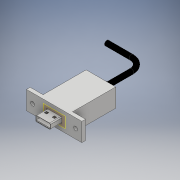
# Autodesk Inventor part: usb head
Saved by Autodesk Inventor 2018 (Build 220112000, 112)
## iProperties
Created: 2017-01-24
Part Number: usb head
Material: Generic
Document SubType Name: Modeling
Designer: shinezackery
Density: 1 g/cm^3
Appearance: Default
Author: shinezackery
Autodesk Inventor part; units mm, degrees
ref_plane "YZ Plane" through (0, 0, 0) normal (1, 0, 0) x (0, 1, 0)
ref_plane "XZ Plane" through (0, 0, 0) normal (0, 1, 0) x (-1, 0, 0)
ref_plane "XY Plane" through (0, 0, 0) normal (0, 0, 1) x (1, 0, 0)
sketch "Sketch1" plane through (0, 0, 0) normal (0, 0, 1) x (1, 0, 0)
  line L0 (0, 0) -> (16.16, 0)
  line L1 (16.16, 0) -> (16.16, 20.88)
  line L2 (16.16, 20.88) -> (13.48, 31.48)
  line L3 (13.48, 31.48) -> (2.68, 31.48)
  line L4 (2.68, 31.48) -> (0, 20.88)
  line L5 (0, 20.88) -> (0, 0)
  point P0 (8.08, 31.48)
  point P1 (8.08, 0)
  dimension "d2" = 16.16
  dimension "d3" = 20.88
  dimension "d4" = 10.8
  dimension "d5" = 10.6
  constraints: 12 end point, 2 horizontal, 2 midpoint, 2 vertical, 1 horizontal alignment, 1 vertical alignment
  measures "d2" distance of L0.start L0.end
  measures "d3" distance of L0.end L1.end
  measures "d4" distance of L2.end L3.end
  measures "d5" vertical distance of L1.end L2.end
extrude "Extrusion1" add sketch "Sketch1" along normal blind 8
chamfer "Chamfer1" distance 1 angle 45 8 edges at (16.16, 10.44, 8) (14.82, 26.18, 8) (14.82, 26.18, 0) (16.16, 10.44, 0) (0, 10.44, 0) (0, 10.44, 8) (1.34, 26.18, 0) (1.34, 26.18, 8)
fillet "Fillet1" radius 0.5 16 edges at (15.16, 10.3778, 8) (13.8043, 26.1178, 8) (14.82, 26.18, 7) (16.16, 10.44, 7) (16.16, 10.44, 1) (15.16, 10.3778, 0) (14.82, 26.18, 1) (13.8043, 26.1178, 0) (1.34, 26.18, 1) (2.3557, 26.1178, 0) (0, 10.44, 1) (1, 10.3778, 0) (1.34, 26.18, 7) (2.3557, 26.1178, 8) (1, 10.3778, 8) (0, 10.44, 7)
fillet "Fillet2" radius 3 7 edges at (0.0381, 20.8753, 6.9842) (0.5, 20.8178, 7.5) (1.0158, 20.7536, 7.9619) (0.0381, 20.8753, 1.0158) (0.5, 20.8178, 0.5) (1.0158, 20.7536, 0.0381) (0, 20.88, 4)
fillet "Fillet3" radius 3 7 edges at (16.1219, 20.8753, 6.9842) (15.66, 20.8178, 7.5) (15.1442, 20.7536, 7.9619) (16.1219, 20.8753, 1.0158) (15.66, 20.8178, 0.5) (15.1442, 20.7536, 0.0381) (16.16, 20.88, 4)
sketch "Sketch2" plane through (0, 0, 8) normal (0, 0, 1) x (1, 0, 0)
  line L0 (4.205, 2.3) -> (11.955, 2.3)
  line L1 (11.955, 2.3) -> (11.955, 17.2)
  line L2 (11.955, 17.2) -> (4.205, 17.2)
  line L3 (4.205, 17.2) -> (4.205, 2.3)
  line L4 (1.2071, 0) -> (14.9529, 0) projected
  point P0 (0, 0)
  point P1 (8.08, 0)
  point P2 (8.08, 2.3)
  dimension "d14" = 7.75
  dimension "d15" = 14.9
  dimension "d16" = 2.3
  constraints: 8 end point, 2 midpoint, 2 parallel, 1 horizontal, 1 perpendicular, 1 vertical alignment
  measures "d14" distance of L1.end L2.end
  measures "d15" distance of L0.end L1.end
  measures "d16" distance between parallel lines of L0 L4
extrude "Extrusion2" cut sketch "Sketch2" against normal blind 0.3
sketch "Sketch4" plane through (1.2071, 0, 0) normal (0, -1, 0) x (1, 0, 0)
  line L0 (0.8729, 1.75) -> (12.8729, 1.75)
  line L1 (12.8729, 1.75) -> (12.8729, 6.25)
  line L2 (12.8729, 6.25) -> (0.8729, 6.25)
  line L3 (0.8729, 6.25) -> (0.8729, 1.75)
  line L4 (0, 8) -> (13.7458, 8) projected
  line L5 (14.9529, 1.2071) -> (14.9529, 6.7929) projected
  point P0 (-1.2071, 0)
  point P1 (6.8729, 6.25)
  point P2 (6.8729, 8)
  point P3 (12.8729, 4)
  point P4 (14.9529, 4)
  dimension "d19" = 12
  dimension "d20" = 4.5
  constraints: 8 end point, 4 midpoint, 3 perpendicular, 1 horizontal, 1 horizontal alignment, 1 vertical alignment
  measures "d19" distance of L1.end L2.end
  measures "d20" distance of L0.end L1.end
extrude "Extrusion3" add sketch "Sketch4" along normal blind 12
fillet "Fillet4" radius 0.75 4 edges at (14.08, -6, 6.25) (14.08, -6, 1.75) (2.08, -6, 6.25) (2.08, -6, 1.75)
sketch "Sketch5" plane through (2.83, 0, 6.25) normal (0, 0, 1) x (1, 0, 0)
  line L0 (7.45, -7) -> (9.45, -7)
  line L1 (9.45, -7) -> (9.45, -5)
  line L2 (9.45, -5) -> (7.45, -5)
  line L3 (7.45, -5) -> (7.45, -7)
  line L4 (3.05, -7) -> (1.05, -7)
  line L5 (1.05, -7) -> (1.05, -5)
  line L6 (1.05, -5) -> (3.05, -5)
  line L7 (3.05, -5) -> (3.05, -7)
  line L8 (10.5, -12) -> (0, -12) projected
  line L9 (-1.6229, 0) -> (12.1229, 0) projected
  line L10 (11.25, -12) -> (11.25, 0) projected
  line L11 (-0.75, 0) -> (-0.75, -12) projected
  line L12 (0, 0) -> (10.5, 0) projected
  line L13 (5.6528, 0) -> (5.6528, -0.9812)
  line L14 (5.6528, -0.9812) -> (5.25, -0.9812)
  line L15 (5.25, -0.9812) -> (5.25, -8.4409)
  line L16 (5.25, -8.4409) -> (5.7498, -8.4409)
  line L17 (5.7498, -8.4409) -> (5.7498, -10.4572)
  line L18 (5.7498, -10.4572) -> (5.25, -10.4572)
  line L19 (5.25, -10.4572) -> (5.25, -12)
  point P0 (-2.83, 0)
  dimension "d24" = 5
  dimension "d25" = 5
  dimension "d26" = 2
  dimension "d27" = 2
  dimension "d28" = 1.8
  dimension "d29" = 1.8
  constraints: 30 end point, 8 perpendicular, 4 parallel, 4 point on line, 2 horizontal, 1 midpoint
  measures "d24" distance between parallel lines of L8 L0
  measures "d25" distance between parallel lines of L9 L2
  measures "d26" distance between parallel lines of L3 L1
  measures "d27" distance between parallel lines of L7 L5
  measures "d28" distance between parallel lines of L10 L1
  measures "d29" distance between parallel lines of L11 L5
extrude "Extrusion4" cut sketch "Sketch5" against normal blind 2.45
sketch "Sketch6" plane through (1.2071, -12, 0) normal (0, -1, 0) x (1, 0, 0)
  arc A0 (0.8729, 2.5) -> (1.6229, 1.75) centre (1.6229, 2.5) ccw projected
  line L0 (1.6229, 1.75) -> (12.1229, 1.75) projected
  arc A1 (12.1229, 1.75) -> (12.8729, 2.5) centre (12.1229, 2.5) ccw projected
  line L1 (12.8729, 2.5) -> (12.8729, 5.5) projected
  arc A2 (12.8729, 5.5) -> (12.1229, 6.25) centre (12.1229, 5.5) ccw projected
  line L2 (12.1229, 6.25) -> (1.6229, 6.25) projected
  arc A3 (1.6229, 6.25) -> (0.8729, 5.5) centre (1.6229, 5.5) ccw projected
  line L3 (0.8729, 5.5) -> (0.8729, 2.5) projected
  line L4 (1.6229, 5.95) -> (12.1229, 5.95)
  arc A4 (12.5729, 5.5) -> (12.1229, 5.95) centre (12.1229, 5.5) ccw
  line L5 (12.5729, 5.5) -> (12.5729, 2.5)
  arc A5 (12.1229, 2.05) -> (12.5729, 2.5) centre (12.1229, 2.5) ccw
  line L6 (12.1229, 2.05) -> (1.6229, 2.05)
  arc A6 (1.1729, 2.5) -> (1.6229, 2.05) centre (1.6229, 2.5) ccw
  line L7 (1.1729, 2.5) -> (1.1729, 5.5)
  arc A7 (1.6229, 5.95) -> (1.1729, 5.5) centre (1.6229, 5.5) ccw
  point P0 (-1.2071, 0)
  dimension "d32" = 0.3
  constraints: 8 end point, 8 point on circle, 4 centre point, 7 other
  measures "d32" distance between parallel lines of L2 L4
extrude "Extrusion5" cut sketch "Sketch6" against normal blind 0.2 contours L4 A4 L5 A5 L6 A6 L7 A7
sketch "Sketch7" plane through (1.2071, -11.8, 0) normal (0, -1, 0) x (1, 0, 0)
  line L0 (1.1729, 2.5) -> (1.1729, 5.5) projected
  line L1 (1.1739, 2.8515) -> (12.5698, 2.8515)
  line L2 (12.1229, 2.05) -> (1.6229, 2.05) projected
  arc A0 (1.6229, 5.95) -> (1.1729, 5.5) centre (1.6229, 5.5) ccw projected
  line L3 (1.6229, 5.95) -> (12.1229, 5.95) projected
  arc A1 (12.5729, 5.5) -> (12.1229, 5.95) centre (12.1229, 5.5) ccw projected
  line L4 (12.5729, 5.5) -> (12.5729, 2.5) projected
  line L5 (12.5719, 2.8515) -> (12.5719, 5.5)
  arc A2 (12.5719, 5.5) -> (12.1229, 5.949) centre (12.1229, 5.5) ccw
  line L6 (12.1229, 5.949) -> (1.6229, 5.949)
  arc A3 (1.6229, 5.949) -> (1.1739, 5.5) centre (1.6229, 5.5) ccw
  line L7 (1.1739, 5.5) -> (1.1739, 2.8515)
  line L8 (12.5698, 2.8515) -> (12.5719, 2.8515)
  point P0 (-1.2071, 0)
  dimension "d35" = 0.8015
  dimension "d36" = 0.001
  constraints: 10 end point, 4 point on circle, 2 centre point, 2 horizontal, 2 perpendicular, 1 point on line, 2 other
  measures "d35" distance between parallel lines of L2 L1
  measures "d36" distance between parallel lines of L6 L3
extrude "Extrusion6" cut sketch "Sketch7" against normal blind 9
sketch "Sketch8" plane through (0, 0, 7.7) normal (0, 0, 1) x (1, 0, 0)
  arc A0 (8.4073, 14.3419) -> (7.8073, 14.3289) centre (8.08, 15.6) ccw
  line L0 (4.205, 17.2) -> (11.955, 17.2) projected
  line L1 (7.8073, 4.1746) -> (7.3073, 4.1746)
  line L2 (8.4073, 4.1746) -> (8.9073, 4.1746)
  line L3 (7.3073, 4.1746) -> (8.08, 2.7708)
  line L4 (8.9073, 4.1746) -> (8.08, 2.7708)
  line L5 (8.4073, 12.3419) -> (9.9118, 11.2001)
  line L6 (8.6051, 12.7918) -> (10.4748, 11.3729)
  line L7 (11.955, 2.3) -> (4.205, 2.3) projected
  arc A1 (10.8703, 10.5763) -> (10.4748, 11.3729) centre (9.8703, 10.5763) ccw
  arc A2 (10.3073, 10.4035) -> (9.9118, 11.2001) centre (9.3073, 10.4035) ccw
  arc A3 (10.3073, 8.7573) -> (10.8703, 8.7573) centre (10.5888, 7.85) ccw
  line L8 (10.3073, 10.4035) -> (10.3073, 8.7573)
  line L9 (10.8703, 10.5763) -> (10.8703, 8.7573)
  line L10 (8.4073, 4.1746) -> (8.4073, 12.3419)
  line L11 (8.4073, 13.1901) -> (8.4073, 14.3419)
  arc A4 (8.4073, 13.1901) -> (8.6051, 12.7918) centre (8.9073, 13.1901) ccw
  line L12 (7.6001, 11.5555) -> (5.4489, 8.7573)
  line L13 (5.4489, 8.7573) -> (5.4489, 6.9)
  line L14 (6.0489, 6.9) -> (6.0489, 8.4673)
  line L15 (6.0489, 8.4673) -> (7.8073, 10.7545)
  line L16 (6.5489, 6.9) -> (6.5489, 5.4)
  line L17 (6.5489, 5.4) -> (4.9489, 5.4)
  line L18 (4.9489, 5.4) -> (4.9489, 6.9)
  line L19 (4.9489, 6.9) -> (5.4489, 6.9)
  line L20 (6.0489, 6.9) -> (6.5489, 6.9)
  line L21 (7.8073, 4.1746) -> (7.8073, 10.7545)
  line L22 (7.8073, 12.165) -> (7.8073, 14.3289)
  arc A5 (7.6001, 11.5555) -> (7.8073, 12.165) centre (6.8073, 12.165) ccw
  point P0 (0, 0)
  point P1 (8.08, 17.2)
  point P2 (10.3073, 10.9)
  constraints: 42 end point, 12 point on circle, 6 centre point, 6 parallel, 6 tangent, 6 vertical, 4 horizontal, 2 collinear, 2 perpendicular, 1 equal radius, 1 midpoint, 1 point on line, 1 vertical alignment
extrude "Extrusion7" add sketch "Sketch8" along normal blind 0.3
sketch "Sketch9" plane through (3.9251, 31.48, 0) normal (0, 1, 0) x (1, 0, 0)
  ellipse E0 centre (0, -7.5) end of major axis (-0.5157, -7.5) minor radius 0.5 (-0.3647, -7.8536) -> (0, -8) ccw projected
  line L0 (8.3098, -8) -> (0, -8) projected
  ellipse E1 centre (8.3098, -7.5) end of major axis (8.8256, -7.5) minor radius 0.5 (8.3098, -8) -> (8.6745, -7.8536) ccw projected
  line L1 (9.4039, -7.1464) -> (8.6745, -7.8536) projected
  ellipse E2 centre (9.0392, -6.7929) end of major axis (9.5549, -6.7929) minor radius 0.5 (9.4039, -7.1464) -> (9.5549, -6.7929) ccw projected
  line L2 (9.5549, -1.2071) -> (9.5549, -6.7929) projected
  ellipse E3 centre (9.0392, -1.2071) end of major axis (9.5549, -1.2071) minor radius 0.5 (9.5549, -1.2071) -> (9.4039, -0.8536) ccw projected
  line L3 (8.6745, -0.1464) -> (9.4039, -0.8536) projected
  ellipse E4 centre (8.3098, -0.5) end of major axis (8.8256, -0.5) minor radius 0.5 (8.6745, -0.1464) -> (8.3098, 0) ccw projected
  line L4 (8.3098, 0) -> (0, 0) projected
  ellipse E5 centre (0, -0.5) end of major axis (-0.5157, -0.5) minor radius 0.5 (0, 0) -> (-0.3647, -0.1464) ccw projected
  line L5 (-1.094, -0.8536) -> (-0.3647, -0.1464) projected
  ellipse E6 centre (-0.7294, -1.2071) end of major axis (-1.2451, -1.2071) minor radius 0.5 (-1.094, -0.8536) -> (-1.2451, -1.2071) ccw projected
  line L6 (-1.2451, -1.2071) -> (-1.2451, -6.7929) projected
  ellipse E7 centre (-0.7294, -6.7929) end of major axis (-1.2451, -6.7929) minor radius 0.5 (-1.2451, -6.7929) -> (-1.094, -7.1464) ccw projected
  line L7 (-0.3647, -7.8536) -> (-1.094, -7.1464) projected
  circle A0 centre (4.1549, -4) radius 3.7
  point P0 (-3.9251, 0)
  point P1 (4.1549, -8)
  point P2 (-1.2451, -4)
  dimension "d73" = 7.4
  constraints: 2 midpoint, 1 centre point, 1 horizontal alignment, 1 vertical alignment, 8 other
  measures "d73" diameter of A0
extrude "Extrusion8" add sketch "Sketch9" along normal blind 8.3 draft -5 contours A0
sketch "Sketch10" plane through (8.08, 39.78, 4) normal (0, 1, 0) x (1, 0, 0)
  circle A0 centre (0, 0) radius 1.95
  point P0 (-8.08, 4)
  dimension "d76" = 3.9
  constraints: 1 centre point
  measures "d76" diameter of A0
extrude "Extrusion9" add sketch "Sketch10" along normal blind 20
sketch "Sketch11" plane through (8.08, 59.78, 4) normal (0, 1, 0) x (1, 0, 0)
  circle A0 centre (0, 0) radius 1.95
  point P0 (-8.08, 4)
  constraints: 1 centre point
ref_plane "Work Plane1" through (0, 0, 4) normal (0, 0, 1) x (1, 0, 0)
sketch "Sketch12" plane through (0, 0, 4) normal (0, 0, 1) x (1, 0, 0)
  line L0 (10.03, 59.78) -> (6.13, 59.78) projected
  line L1 (8.08, 59.78) -> (8.08, 59.78)
  line L2 (-1.92, 69.78) -> (-21.92, 69.78)
  arc A0 (8.08, 59.78) -> (-1.92, 69.78) centre (-1.92, 59.78) ccw
  point P0 (0, 0)
  point P1 (8.08, 69.78)
  dimension "d79" = 10
  dimension "d80" = 30
  dimension "d81" = 10
  constraints: 4 end point, 2 point on circle, 2 point on line, 2 tangent, 1 centre point, 1 midpoint, 1 perpendicular, 1 vertical
  measures "d79" distance of L1.start point (8.08, 69.78)
  measures "d80" distance of point (8.08, 69.78) L2.end
  measures "d81" radius of A0
sweep "Sweep1" add profiles "Sketch11" path "Sketch12" path curves A0 L2
ref_plane "Work Plane2" through (1.2071, -3, 0) normal (0, -1, 0) x (1, 0, 0)
sketch "Sketch13" plane through (1.2071, -3, 0) normal (0, -1, 0) x (1, 0, 0)
  point P0 (-1.2071, 0)
sketch "Sketch14" plane through (1.2071, -3, 0) normal (0, -1, 0) x (1, 0, 0)
  line L0 (-1.2071, 1.2071) -> (-1.2071, 6.7929) projected
  line L1 (-1.2071, 4) -> (14.9529, 4)
  line L2 (14.9529, 6.7929) -> (14.9529, 1.2071) projected
  line L3 (6.8729, 4) -> (6.8729, 7.9846)
  line L4 (6.8729, 4) -> (6.8729, 0)
  line L5 (13.0729, 1.55) -> (0.6729, 1.55)
  line L6 (0.6729, 1.55) -> (0.6729, 6.45)
  line L7 (0.6729, 6.45) -> (13.0729, 6.45)
  line L8 (13.0729, 6.45) -> (13.0729, 1.55)
  line L9 (13.0729, 1.55) -> (0.6729, 6.45) construction
  line L10 (0.6729, 1.55) -> (13.0729, 6.45) construction
  line L11 (29.3729, -3.5) -> (-15.6271, -3.5)
  line L12 (-15.6271, -3.5) -> (-15.6271, 11.5)
  line L13 (-15.6271, 11.5) -> (29.3729, 11.5)
  line L14 (29.3729, 11.5) -> (29.3729, -3.5)
  line L15 (29.3729, -3.5) -> (-15.6271, 11.5) construction
  line L16 (-15.6271, -3.5) -> (29.3729, 11.5) construction
  point P0 (-1.2071, 0)
  dimension "d85" = 12.4
  dimension "d86" = 4.9
  dimension "d87" = 45
  dimension "d88" = 15
  constraints: 30 end point, 7 midpoint, 4 parallel, 2 horizontal, 2 perpendicular, 2 vertical
  measures "d85" distance of L6.end L7.end
  measures "d86" distance of L5.end L6.end
  measures "d87" distance of L12.end L13.end
  measures "d88" distance of L11.end L12.end
extrude "Extrusion10" add sketch "Sketch14" against normal blind 3
sketch "Sketch15" plane through (1.2071, 0, 0) normal (0, 1, 0) x (1, 0, 0)
  line L0 (-15.6271, -11.5) -> (29.3729, -11.5) projected
  line L1 (29.3729, 3.5) -> (-15.6271, 3.5) projected
  line L2 (29.3729, -11.5) -> (-15.6271, 3.5)
  line L3 (29.3729, 3.5) -> (-15.6271, -11.5)
  line L4 (-5.1271, 3.5) -> (18.8729, 3.5)
  line L5 (18.8729, 3.5) -> (18.8729, -11.5)
  line L6 (18.8729, -11.5) -> (-5.1271, -11.5)
  line L7 (-5.1271, -11.5) -> (-5.1271, 3.5)
  line L8 (-5.1271, 3.5) -> (18.8729, -11.5) construction
  line L9 (18.8729, 3.5) -> (-5.1271, -11.5) construction
  line L10 (-1.6271, 0.5) -> (15.3729, 0.5)
  line L11 (15.3729, 0.5) -> (15.3729, -8.5)
  line L12 (15.3729, -8.5) -> (-1.6271, -8.5)
  line L13 (-1.6271, -8.5) -> (-1.6271, 0.5)
  line L14 (-1.6271, 0.5) -> (15.3729, -8.5) construction
  line L15 (15.3729, 0.5) -> (-1.6271, -8.5) construction
  point P0 (-1.2071, 0)
  point P1 (6.8729, -4)
  dimension "d91" = 24
  dimension "d92" = 17
  dimension "d93" = 9
  constraints: 28 end point, 5 midpoint, 4 parallel, 2 horizontal, 2 perpendicular, 1 point on line
  measures "d91" distance of L5.end L6.end
  measures "d92" distance of L11.end L12.end
  measures "d93" distance of L10.end L11.end
extrude "Extrusion11" add sketch "Sketch15" along normal blind 35 contours L7 L3 L13 L12 L11 L2 L5 L0 | L7 L2 L13 L3 | L7 L1 L5 L3 L11 L10 L13 L2 | L2 L11 L3 L5
sketch "Sketch16" plane through (1.2071, -3, 0) normal (0, -1, 0) x (1, 0, 0)
  circle A0 centre (-10.6271, 4) radius 1.6
  line L0 (-5.1271, 11.5) -> (18.8729, 11.5) projected
  line L1 (6.8729, 11.5) -> (6.8729, -3.5)
  line L2 (18.8729, -3.5) -> (-5.1271, -3.5) projected
  circle A1 centre (24.3729, 4) radius 1.6
  line L3 (-15.6271, -3.5) -> (-15.6271, 11.5) projected
  point P0 (-1.2071, 0)
  dimension "d96" = 3.2
  dimension "d97" = 5
  constraints: 2 centre point, 2 end point, 2 midpoint, 1 symmetric about line, 1 other
  measures "d96" diameter of A0
  measures "d97" distance from line of A0.centre L3
extrude "Extrusion12" cut sketch "Sketch16" against normal blind 3
body "Solid1"
